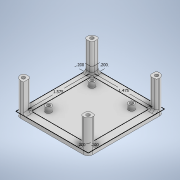
# Autodesk Inventor part: SensorHousing
Saved by Autodesk Inventor 2020 (Build 240168000, 168)
## iProperties
Created: 2022-06-20
Part Number: SensorHousing
Material: Generic
Document SubType Name: Modeling
Designer: Beaucage
Density: 1 g/cm^3
Appearance: Default
Author: Beaucage
Autodesk Inventor part; units mm, degrees
ref_plane "YZ Plane" through (0, 0, 0) normal (1, 0, 0) x (0, 1, 0)
ref_plane "XZ Plane" through (0, 0, 0) normal (0, 1, 0) x (-1, 0, 0)
ref_plane "XY Plane" through (0, 0, 0) normal (0, 0, 1) x (1, 0, 0)
sketch "Sketch1" plane through (0, 0, 0) normal (0, 1, 0) x (-1, 0, 0)
  line L0 (0, 0) -> (5.08, 0)
  line L1 (5.08, 0) -> (5.08, -5.08)
  line L2 (5.08, -5.08) -> (0, -5.08)
  line L3 (0, -5.08) -> (0, 0)
  line L4 (5.08, -5.08) -> (42.545, -5.08)
  line L5 (42.545, -5.08) -> (42.545, -45.085)
  line L6 (42.545, -45.085) -> (5.08, -45.085)
  line L7 (5.08, -45.085) -> (5.08, -5.08)
  line L8 (42.545, -45.085) -> (47.625, -45.085)
  line L9 (47.625, -45.085) -> (47.625, -50.165)
  line L10 (47.625, -50.165) -> (42.545, -50.165)
  line L11 (42.545, -50.165) -> (42.545, -45.085)
  line L12 (47.625, -50.165) -> (0, -50.165)
  line L13 (0, -50.165) -> (0, 0)
  line L14 (0, 0) -> (47.625, 0)
  line L15 (47.625, 0) -> (47.625, -50.165)
  line L16 (42.545, -5.08) -> (47.625, -5.08)
  line L17 (47.625, -5.08) -> (47.625, 0)
  line L18 (47.625, 0) -> (42.545, 0)
  line L19 (42.545, 0) -> (42.545, -5.08)
  line L20 (5.08, -45.085) -> (0, -45.085)
  line L21 (0, -45.085) -> (0, -50.165)
  line L22 (0, -50.165) -> (5.08, -50.165)
  line L23 (5.08, -50.165) -> (5.08, -45.085)
  dimension "d0" = 5.08
  dimension "d1" = 5.08
  dimension "d2" = 37.465
  dimension "d3" = 40.005
  dimension "d4" = 5.08
  dimension "d5" = 5.08
  constraints: 48 end point, 12 parallel, 6 horizontal, 6 perpendicular
  measures "d0" distance of L1.end L2.end
  measures "d1" distance of L0.end L1.end
  measures "d2" distance of L5.end L6.end
  measures "d3" distance of L4.end L5.end
  measures "d4" distance of L9.end L10.end
  measures "d5" distance of L8.end L9.end
extrude "Extrusion1" add sketch "Sketch1" against normal blind 2.54
extrude "Extrusion2" add sketch "Sketch1" along normal blind 19.05 contours L0 L1 L2 L3 | L14 L15 L16 L19 | L20 L23 L12 L13 | L8 L9 L10 L11
sketch "Sketch2" plane through (0, 0, 0) normal (0, 1, 0) x (1, 0, 0)
  line L0 (-47.625, 45.085) -> (-47.625, 5.08) projected
  line L1 (-47.625, 25.0825) -> (0, 25.0825)
  line L2 (0, 25.0825) -> (-23.8125, 25.0825)
  line L3 (-10.795, 10.795) -> (-36.83, 10.795)
  line L4 (-36.83, 10.795) -> (-36.83, 39.37)
  line L5 (-36.83, 39.37) -> (-10.795, 39.37)
  line L6 (-10.795, 39.37) -> (-10.795, 10.795)
  line L7 (-10.795, 10.795) -> (-36.83, 39.37) construction
  line L8 (-36.83, 10.795) -> (-10.795, 39.37) construction
  circle A0 centre (-36.83, 10.795) radius 1.905
  circle A1 centre (-36.83, 39.37) radius 1.905
  circle A2 centre (-10.795, 39.37) radius 1.905
  circle A3 centre (-10.795, 10.795) radius 1.905
  point P0 (0, 0)
  dimension "d10" = 26.035
  dimension "d11" = 28.575
  dimension "d12" = 3.81
  dimension "d13" = 3.81
  dimension "d14" = 3.81
  dimension "d15" = 3.81
  constraints: 16 end point, 4 centre point, 4 coincident, 4 midpoint, 2 horizontal, 2 parallel, 1 perpendicular
  measures "d10" distance of L4.end L5.end
  measures "d11" distance of L3.end L4.end
  measures "d12" diameter of A0
  measures "d13" diameter of A1
  measures "d14" diameter of A2
  measures "d15" diameter of A3
extrude "Extrusion3" add sketch "Sketch2" along normal blind 3.175 contours A0 L3 L4 | L4 L3 A0 | A1 L5 L4 | L4 L5 A1 | A2 L5 L6 | L6 L5 A2 | A3 L3 L6 | L6 L3 A3
sketch "Sketch3" plane through (-36.83, 3.175, -10.795) normal (0, 1, 0) x (1, 0, 0)
  circle A0 centre (26.035, 0) radius 1.905 projected
  circle A1 centre (26.035, 28.575) radius 1.905 projected
  circle A2 centre (0, 28.575) radius 1.905 projected
  point P0 (36.83, -10.795)
  point P1 (0, 0)
  constraints: 3 coincident
hole "Hole1" at (-36.83, 3.175, -10.795) at (-36.83, 3.175, -39.37) at (-10.795, 3.175, -39.37) at (-10.795, 3.175, -10.795) direction (0, -1, 0) diameter 2.2606 depth 5.6896
sketch "Sketch4" plane through (0, 19.05, 0) normal (0, 1, 0) x (1, 0, 0)
  line L0 (-47.625, 50.165) -> (-47.625, 45.085) projected
  line L1 (-47.625, 50.165) -> (-45.085, 50.165)
  line L2 (-45.085, 50.165) -> (-45.085, 47.625)
  line L3 (-45.085, 47.625) -> (-47.625, 47.625)
  line L4 (-47.625, 47.625) -> (-47.625, 50.165)
  line L5 (-47.625, 0) -> (-47.625, 50.165) projected
  line L6 (-47.625, 0) -> (-45.085, 0)
  line L7 (-45.085, 0) -> (-45.085, 2.54)
  line L8 (-45.085, 2.54) -> (-47.625, 2.54)
  line L9 (-47.625, 2.54) -> (-47.625, 0)
  line L10 (0, 0) -> (-47.625, 0) projected
  line L11 (0, 0) -> (-2.54, 0)
  line L12 (-2.54, 0) -> (-2.54, 2.54)
  line L13 (-2.54, 2.54) -> (0, 2.54)
  line L14 (0, 2.54) -> (0, 0)
  line L15 (-47.625, 50.165) -> (0, 50.165) projected
  line L16 (0, 50.165) -> (-2.54, 50.165)
  line L17 (-2.54, 50.165) -> (-2.54, 47.625)
  line L18 (-2.54, 47.625) -> (0, 47.625)
  line L19 (0, 47.625) -> (0, 50.165)
  dimension "d25" = 2.54
  dimension "d26" = 2.54
  dimension "d27" = 2.54
  constraints: 32 end point, 8 parallel, 4 horizontal, 4 perpendicular, 4 point on line
  measures "d25" distance of L2.end L3.end
  measures "d26" distance of L7.end L6.end
  measures "d27" distance of L12.end L13.end
hole "Hole2" at (-45.085, 19.05, -47.625) at (-2.54, 19.05, -47.625) at (-2.54, 19.05, -2.54) at (-45.085, 19.05, -2.54) direction (0, -1, 0) diameter 2.2606 depth 5.6896
fillet "Fillet1" radius 3.175 4 edges at (-47.625, 8.255, -50.165) (-47.625, 8.255, 0) (0, 8.255, -50.165) (0, 8.255, 0)
fillet "Fillet2" radius 1.5875 19 edges at (-45.085, 0, -45.085) (-42.545, 0, -47.625) (-42.545, 0, -2.54) (-2.54, 0, -45.085) (-45.085, 0, -5.08) (-5.08, 0, -47.625) (-2.54, 0, -5.08) (-5.08, 0, -2.54) (-5.08, 9.525, -45.085) (-5.08, 9.525, -5.08) (-5.08, 9.525, 0) (0, 9.525, -5.08) (-42.545, 9.525, -5.08) (-47.625, 9.525, -5.08) (-47.625, 9.525, -45.085) (-42.545, 9.525, -50.165) (-5.08, 9.525, -50.165) (0, 9.525, -45.085) (-42.545, 9.525, -45.085)
body "Solid1"
